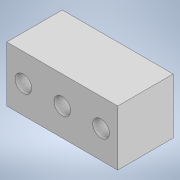
# Autodesk Inventor part: 指下
Saved by Autodesk Inventor 2022 (Build 260153070, 153G)
## iProperties
Created: 2022-10-10
Part Number: 指下
Material: 一般
Document SubType Name: Modeling
Designer: hirok
Density: 1 g/cm^3
Appearance: 既定
Author: hirok
Autodesk Inventor part; units mm, degrees
ref_plane "YZ Plane" through (0, 0, 0) normal (1, 0, 0) x (0, 1, 0)
ref_plane "XZ Plane" through (0, 0, 0) normal (0, 1, 0) x (-1, 0, 0)
ref_plane "XY Plane" through (0, 0, 0) normal (0, 0, 1) x (1, 0, 0)
sketch "スケッチ1" plane through (0, 0, 0) normal (0, 0, 1) x (1, 0, 0)
  line L0 (0, 0) -> (20, 0)
  line L1 (20, 0) -> (20, 10)
  line L2 (20, 10) -> (0, 10)
  line L3 (0, 10) -> (0, 0)
  dimension "d0" = 20
  dimension "d1" = 10
  constraints: 8 end point, 2 parallel, 1 horizontal, 1 perpendicular
  measures "d0" distance of L1.end L2.end
  measures "d1" distance of L0.end L1.end
extrude "押し出し1" add sketch "スケッチ1" along normal blind 10
sketch "スケッチ3" plane through (0, 0, 10) normal (0, 0, 1) x (1, 0, 0)
  line L0 (20, 10) -> (0, 10) projected
  point P0 (0, 0)
  point P1 (10, 5)
  dimension "d13" = 5
  measures "d13" distance from line of point (10, 5) L0
hole "穴2" at (10, 5, 10) direction (0, 0, -1) diameter 3 end through all
sketch "スケッチ4" plane through (0, 0, 10) normal (0, 0, 1) x (1, 0, 0)
  line L0 (0, 10) -> (0, 0) projected
  line L1 (20, 0) -> (20, 10) projected
  point P0 (3, 5)
  point P1 (17, 5)
  dimension "d21" = 3
  dimension "d22" = 3
  measures "d21" distance from line of L0 point (3, 5)
  measures "d22" distance from line of L1 point (17, 5)
hole "穴3" at (3, 5, 10) at (17, 5, 10) direction (0, 0, -1) diameter 3 end through all
